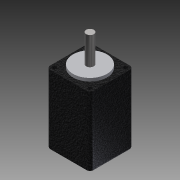
# Autodesk Inventor part: NEMA11
Saved by Autodesk Inventor 2014 SP2 (Build 180246200, 246)
## iProperties
Created: 2015-11-29
Part Number: NEMA11
Material: Generic
Document SubType Name: Modeling
Designer: schrluka
Density: 1 g/cm^3
Appearance: Default
Author: schrluka
Autodesk Inventor part; units mm, degrees
ref_plane "YZ Plane" through (0, 0, 0) normal (1, 0, 0) x (0, 1, 0)
ref_plane "XZ Plane" through (0, 0, 0) normal (0, 1, 0) x (-1, 0, 0)
ref_plane "XY Plane" through (0, 0, 0) normal (0, 0, 1) x (1, 0, 0)
sketch "Sketch1" plane through (0, 0, 0) normal (0, 0, 1) x (1, 0, 0)
  line L0 (-14.1, -14.1) -> (14.1, -14.1)
  line L1 (14.1, -14.1) -> (14.1, 14.1)
  line L2 (14.1, 14.1) -> (-14.1, 14.1)
  line L3 (-14.1, 14.1) -> (-14.1, -14.1)
  line L4 (-14.1, -14.1) -> (14.1, 14.1) construction
  line L5 (14.1, -14.1) -> (-14.1, 14.1) construction
  point P0 (0, 0)
  dimension "d0" = 28.2
  dimension "d1" = 28.2
  constraints: 12 end point, 2 midpoint, 2 parallel, 1 horizontal, 1 perpendicular
  measures "d0" distance of L2.end L1.end
  measures "d1" distance of L1.end L0.end
extrude "Extrusion1" add sketch "Sketch1" along normal blind 45
sketch "Sketch2" plane through (0, 0, 45) normal (0, 0, 1) x (1, 0, 0)
  circle A0 centre (0, 0) radius 11
  dimension "d4" = 22
  constraints: 1 centre point, 1 coincident
  measures "d4" diameter of A0
extrude "Extrusion2" add sketch "Sketch2" along normal blind 2
sketch "Sketch3" plane through (0, 0, 47) normal (0, 0, 1) x (1, 0, 0)
  circle A0 centre (0, 0) radius 11 projected
  circle A1 centre (0, 0) radius 2.5
  dimension "d7" = 5
  constraints: 1 centre point, 1 coincident
  measures "d7" diameter of A1
extrude "Extrusion3" add sketch "Sketch3" along normal blind 18 contours A1
sketch "Sketch4" plane through (0, 0, 45) normal (0, 0, 1) x (1, 0, 0)
  circle A0 centre (0, 0) radius 11 projected
  point P0 (-11.5, 11.5)
  point P1 (11.5, 11.5)
  point P2 (11.5, -11.5)
  point P3 (-11.5, -11.5)
  dimension "d10" = 11.5
  dimension "d11" = 11.5
  dimension "d12" = 11.5
  dimension "d13" = 11.5
  dimension "d14" = 11.5
  dimension "d15" = 11.5
  dimension "d16" = 11.5
  dimension "d17" = 11.5
  measures "d10" horizontal distance of A0.centre point (-11.5, 11.5)
  measures "d11" horizontal distance of point (11.5, 11.5) A0.centre
  measures "d12" horizontal distance of point (11.5, -11.5) A0.centre
  measures "d13" horizontal distance of point (-11.5, -11.5) A0.centre
  measures "d14" horizontal distance of point (-11.5, -11.5) A0.centre
  measures "d15" horizontal distance of point (11.5, -11.5) A0.centre
  measures "d16" horizontal distance of A0.centre point (11.5, 11.5)
  measures "d17" horizontal distance of A0.centre point (-11.5, 11.5)
hole "Hole1" at (-11.5, 11.5, 45) at (11.5, 11.5, 45) at (11.5, -11.5, 45) at (-11.5, -11.5, 45) direction (0, 0, -1) diameter 2.5 depth 4.5 tip angle 118
fillet "Fillet1" radius 2.5 4 edges at (-14.1, 14.1, 22.5) (14.1, 14.1, 22.5) (14.1, -14.1, 22.5) (-14.1, -14.1, 22.5)
fillet "Fillet2" radius 1 8 edges at (-13.3678, 13.3678, 0) (-14.1, 0, 0) (-13.3678, -13.3678, 0) (0, -14.1, 0) (13.3678, -13.3678, 0) (14.1, 0, 0) (13.3678, 13.3678, 0) (0, 14.1, 0)
body "Solid1"
